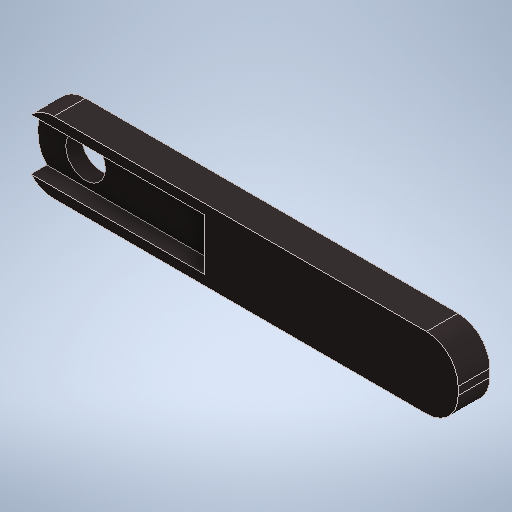
# Autodesk Inventor part: Servo Arm
Saved by Autodesk Inventor 2025.4 (Build 294407000, 407)
## iProperties
Created: 2026-05-20
Part Number: Servo Arm
Material: Generic
Document SubType Name: Modeling
Designer: lenovo
Density: 1 g/cm^3
Appearance: Default(1)
Author: lenovo
Autodesk Inventor part; units mm, degrees
ref_plane "YZ Plane" through (0, 0, 0) normal (1, 0, 0) x (0, 1, 0)
ref_plane "XZ Plane" through (0, 0, 0) normal (0, 1, 0) x (-1, 0, 0)
ref_plane "XY Plane" through (0, 0, 0) normal (0, 0, 1) x (1, 0, 0)
sketch "Sketch1" plane through (0, 0, 0) normal (0, 0, 1) x (1, 0, 0)
  line L0 (-27.5, -4.5) -> (27.5, -4.5)
  line L1 (27.5, -4.5) -> (27.5, 4.5)
  line L2 (27.5, 4.5) -> (-27.5, 4.5)
  line L3 (-27.5, 4.5) -> (-27.5, -4.5)
  line L4 (-27.5, -4.5) -> (27.5, 4.5) construction
  line L5 (27.5, -4.5) -> (-27.5, 4.5) construction
  point P0 (0, 0)
  dimension "d0" = 55
  dimension "d1" = 9
  constraints: 12 end point, 2 midpoint, 2 parallel, 1 horizontal, 1 perpendicular
  measures "d0" distance of L2.end L1.end
  measures "d1" distance of L1.end L0.end
extrude "Extrusion1" add sketch "Sketch1" along normal mid plane 4
sketch "Sketch2" plane through (0, 0, 2) normal (0, 0, 1) x (1, 0, 0)
  line L0 (-27.5, 4.5) -> (-27.5, -4.5) projected
  line L1 (-27.5, -3.25) -> (-4.5, -3.25)
  line L2 (-4.5, -3.25) -> (-4.5, 3.25)
  line L3 (-4.5, 3.25) -> (-27.5, 3.25)
  line L4 (-27.5, 3.25) -> (-27.5, -3.25)
  point P0 (0, 0)
  point P1 (-4.5, 0)
  dimension "d4" = 23
  dimension "d5" = 6.5
  constraints: 8 end point, 2 parallel, 1 horizontal, 1 horizontal alignment, 1 midpoint, 1 perpendicular, 1 point on line
  measures "d4" distance of L3.end L2.end
  measures "d5" distance of L2.end L1.end
extrude "Extrusion2" cut sketch "Sketch2" against normal blind 2
sketch "Sketch3" plane through (0, 0, 0) normal (0, 0, 1) x (1, 0, 0)
  circle A0 centre (-21.5, 0) radius 2.5
  line L0 (-27.5, -3.25) -> (-27.5, 3.25) projected
  point P0 (0, 0)
  dimension "d8" = 5
  dimension "d13" = 6
  constraints: 1 centre point, 1 horizontal alignment
  measures "d8" diameter of A0
  measures "d13" distance from line of L0 A0.centre
extrude "Extrusion3" cut sketch "Sketch3" against normal blind 2
fillet "Fillet1" radius 4 2 edges at (27.5, 4.5, 0) (27.5, -4.5, 0)
fillet "Fillet2" radius 4 2 edges at (-27.5, 4.5, 0) (-27.5, -4.5, 0)
body "Solid1"
